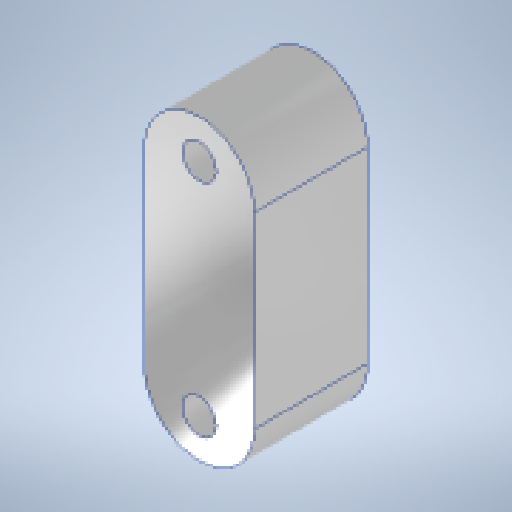
# Autodesk Inventor part: link1part2
Saved by Autodesk Inventor 2024 (Build 280153000, 153)
## iProperties
Created: 2025-02-07
Part Number: link1part2
Material: アルミニウム 6061
Document SubType Name: Modeling
Designer: tanoue_kota
Mass: 6.303 g
Surface Area: 13.1583 cm^2
Volume: 2.33444 cm^3
Density: 2.7 g/cm^3
Appearance: アルミニウム - フラット
Author: tanoue_kota
Autodesk Inventor part; units mm, degrees
ref_plane "YZ Plane" through (0, 0, 0) normal (1, 0, 0) x (0, 1, 0)
ref_plane "XZ Plane" through (0, 0, 0) normal (0, 1, 0) x (-1, 0, 0)
ref_plane "XY Plane" through (0, 0, 0) normal (0, 0, 1) x (1, 0, 0)
sketch "スケッチ1" plane through (0, 0, 0) normal (0, 0, 1) x (1, 0, 0)
  line L0 (0, 0) -> (10, 0)
  line L1 (10, 0) -> (10, 27)
  line L2 (10, 27) -> (0, 27)
  line L3 (0, 27) -> (0, 0)
  dimension "d0" = 27
  dimension "d1" = 10
  constraints: 8 end point, 2 parallel, 1 horizontal, 1 perpendicular
  measures "d0" distance of L0.end L1.end
  measures "d1" distance of L1.end L2.end
extrude "押し出し1" add sketch "スケッチ1" along normal blind 10.273
sketch "スケッチ2" plane through (0, 0, 10.273) normal (0, 0, 1) x (1, 0, 0)
  line L0 (0, 27) -> (0, 0) projected
  line L1 (0, 13.5) -> (10, 13.5)
  line L2 (10, 0) -> (10, 27) projected
  line L3 (10, 27) -> (0, 27) projected
  line L4 (5, 27) -> (5, 0)
  line L5 (0, 0) -> (10, 0) projected
  line L6 (0, 27) -> (10, 27)
  point P0 (5, 23.5)
  point P1 (5, 3.5)
  dimension "d4" = 10
  constraints: 6 end point, 4 midpoint, 1 point on line, 1 symmetric about line
  measures "d4" distance from line of L1 point (5, 23.5)
hole "穴1" at (5, 23.5, 10.273) at (5, 3.5, 10.273) direction (0, 0, -1) diameter 3.1 end through all
fillet "フィレット1" radius 5 4 edges at (0, 27, 5.1365) (10, 27, 5.1365) (10, 0, 5.1365) (0, 0, 5.1365)
